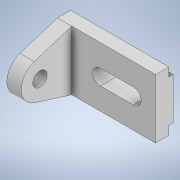
# Autodesk Inventor part: 2.4
Saved by Autodesk Inventor 2022 (Build 260153000, 153)
## iProperties
Created: 2023-04-17
Part Number: 2.4
Material: Genérico
Document SubType Name: Modeling
Designer: jpjoa
Density: 1 g/cm^3
Appearance: Padrão
Author: jpjoa
Autodesk Inventor part; units mm, degrees
ref_plane "YZ Plane" through (0, 0, 0) normal (1, 0, 0) x (0, 1, 0)
ref_plane "XZ Plane" through (0, 0, 0) normal (0, 1, 0) x (-1, 0, 0)
ref_plane "XY Plane" through (0, 0, 0) normal (0, 0, 1) x (1, 0, 0)
sketch "Esboço1" plane through (0, 0, 0) normal (0, 0, 1) x (1, 0, 0)
  line L0 (0, 0) -> (89, 0)
  line L1 (89, 0) -> (89, 54)
  line L2 (89, 54) -> (0, 54)
  line L3 (0, 54) -> (0, 0)
  line L4 (13, 46) -> (89, 46)
  line L5 (89, 8) -> (13, 8)
  line L6 (13, 0) -> (13, 54)
  line L7 (39, 27) -> (69, 27) construction
  line L8 (39, 20) -> (69, 20)
  line L9 (69, 34) -> (39, 34)
  arc A0 (39, 34) -> (39, 20) centre (39, 27) ccw
  arc A1 (69, 20) -> (69, 34) centre (69, 27) ccw
  point P0 (54, 27)
  point P1 (89, 27)
  dimension "d0" = 89
  dimension "d1" = 54
  dimension "d2" = 38
  dimension "d3" = 8
  dimension "d4" = 13
  dimension "d5" = 30
  dimension "d6" = 14
  dimension "d8" = 20
  constraints: 22 end point, 6 perpendicular, 6 point on line, 4 point on circle, 4 tangent, 2 centre point, 2 horizontal, 2 midpoint, 1 horizontal alignment, 1 parallel
  measures "d0" distance of L0.start L0.end
  measures "d1" distance of L0.end L1.end
  measures "d2" distance between parallel lines of L5 L4
  measures "d3" distance between parallel lines of L0 L5
  measures "d4" distance between parallel lines of L3 L6
  measures "d5" distance of L7.start L7.end
  measures "d6" diameter of A1
  measures "d8" distance from line of L1 L7.end
extrude "Extrusão1" add sketch "Esboço1" against normal blind 12 contours L3 L2 L6 L0 | L6 L5 L1 L0 | L2 L1 L4 L6
extrude "Extrusão2" add sketch "Esboço1" against normal blind 16 contours L6 L4 L1 L5
extrude "Extrusão3" add sketch "Esboço1" along normal blind 46 contours L3 L2 L6 L0
sketch "Esboço2" plane through (13, 0, 0) normal (1, 0, 0) x (0, 0, -1)
  circle A0 centre (-29, 27) radius 17
  circle A1 centre (-29, 27) radius 6.5
  line L0 (0, 0) -> (0, 54) projected
  line L1 (0, 54) -> (-46, 54) projected
  line L2 (0, 54) -> (-34.1255, 43.2089)
  line L3 (0, 54) -> (0, 0) projected
  line L4 (0, 0) -> (-34.1255, 10.7911)
  line L5 (0, 0) -> (12, 0) projected
  line L6 (0, 0) -> (-46, 0)
  line L7 (-46, 54) -> (-46, 0) projected
  line L8 (-46, 0) -> (-46, 54)
  line L9 (-46, 54) -> (0, 54)
  line L10 (12, 54) -> (-46, 54) projected
  point P0 (-46, 27)
  dimension "d15" = 34
  dimension "d16" = 13
  dimension "d17" = 29
  dimension "d18" = 27
  constraints: 10 end point, 3 collinear, 2 centre point, 2 point on circle, 2 tangent, 1 concentric
  measures "d15" diameter of A0
  measures "d16" diameter of A1
  measures "d17" distance from line of L0 A0.centre
  measures "d18" distance from line of L1 A0.centre
extrude "Extrusão4" cut sketch "Esboço2" against normal up to surface (13 mm away) contours A0 L7 L1 L2 | L4 L6 L7 A0 | A1
